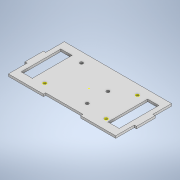
# Autodesk Inventor part: Level2 (Arduino)
Saved by Autodesk Inventor 2020 (Build 240168000, 168)
## iProperties
Created: 2020-01-30
Part Number: Level2 (Arduino)
Material: Generic
Document SubType Name: Modeling
Designer: jelte
Density: 1 g/cm^3
Appearance: Default
Mass: 27.7069 g
Surface Area: 213.533 cm^2
Volume: 27.7069 cm^3
Author: jelte
Autodesk Inventor part; units mm, degrees
ref_plane "YZ Plane" through (0, 0, 0) normal (1, 0, 0) x (0, 1, 0)
ref_plane "XZ Plane" through (0, 0, 0) normal (0, 1, 0) x (-1, 0, 0)
ref_plane "XY Plane" through (0, 0, 0) normal (0, 0, 1) x (1, 0, 0)
sketch "Sketch1" plane through (0, 0, 0) normal (0, 1, 0) x (-1, 0, 0)
  line L0 (71.1097, -38.0648) -> (71.1097, -13.0648)
  line L1 (71.1097, -13.0648) -> (74.1097, -13.0648)
  line L2 (74.1097, -13.0648) -> (74.1097, 11.9352)
  line L3 (74.1097, 11.9352) -> (71.1097, 11.9352)
  line L4 (71.1097, 11.9352) -> (71.1097, 36.9352)
  line L5 (-72.8903, -38.0648) -> (-72.8903, -13.0648)
  line L6 (-72.8903, 36.9352) -> (-72.8903, 11.9352)
  line L7 (-72.8903, -13.0648) -> (-75.8903, -13.0648)
  line L8 (-75.8903, -13.0648) -> (-75.8903, 11.9352)
  line L9 (-75.8903, 11.9352) -> (-72.8903, 11.9352)
  line L10 (71.1097, -38.0648) -> (-72.8903, -38.0648)
  line L11 (71.1097, 36.9352) -> (-72.8903, 36.9352)
  point P0 (0, 0)
  constraints: 24 end point, 5 perpendicular, 3 horizontal, 2 vertical
extrude "Extrusion1" add sketch "Sketch1" along normal blind 3
sketch "Sketch2" plane through (0, 3, 0) normal (0, 1, 0) x (1, 0, 0)
  line L0 (-74.1097, 13.0648) -> (-74.1097, -11.9352) projected
  line L1 (75.8903, -11.9352) -> (75.8903, 13.0648) projected
  line L2 (-71.1097, -36.9352) -> (72.8903, -36.9352) projected
  line L3 (-24.1097, -36.9352) -> (25.8903, -36.9352)
  line L4 (25.8903, -36.9352) -> (25.8903, -33.9352)
  line L5 (25.8903, -33.9352) -> (-24.1097, -33.9352)
  line L6 (-24.1097, -33.9352) -> (-24.1097, -36.9352)
  line L7 (72.8903, 38.0648) -> (-71.1097, 38.0648) projected
  point P0 (0, 0)
  dimension "d13" = 50
  dimension "d14" = 3
  constraints: 8 end point, 2 parallel, 1 horizontal, 1 perpendicular, 1 point on line
  measures "d13" distance of L4.end L5.end
  measures "d14" distance of L3.end L4.end
extrude "Extrusion2" cut sketch "Sketch2" against normal blind 30
sketch "Sketch3" plane through (0, 3, 0) normal (0, 1, 0) x (1, 0, 0)
  line L0 (-71.1097, -36.9352) -> (-24.1097, -36.9352) projected
  line L1 (-74.1097, 13.0648) -> (-74.1097, -11.9352) projected
  line L2 (-54.9097, 25.4648) -> (-64.9114, 25.4648)
  line L3 (-64.9114, 25.4648) -> (-64.9114, -24.8352)
  line L4 (-64.9114, -24.8352) -> (-54.9097, -24.8352)
  line L5 (-54.9097, -24.8352) -> (-54.9097, 25.4648)
  line L6 (56.6903, 25.4648) -> (66.6903, 25.4648)
  line L7 (66.6903, 25.4648) -> (66.6903, -24.8352)
  line L8 (66.6903, -24.8352) -> (56.6903, -24.8352)
  line L9 (56.6903, -24.8352) -> (56.6903, 25.4648)
  circle A0 centre (-34.6697, 22.9248) radius 2
  circle A1 centre (-35.9397, -22.2952) radius 2
  circle A2 centre (40.2603, 22.9248) radius 2
  circle A3 centre (46.6103, -22.2952) radius 2
  line L10 (-49.9097, 28.4648) -> (51.6903, 28.4648)
  line L11 (51.6903, 28.4648) -> (51.6903, 33.4648)
  line L12 (51.6903, 33.4648) -> (-49.9097, 33.4648)
  line L13 (-49.9097, 33.4648) -> (-49.9097, 28.4648)
  point P0 (0, 0)
  dimension "d32" = 4
  dimension "d35" = 4
  dimension "d38" = 4
  dimension "d39" = 4
  constraints: 24 end point, 6 parallel, 4 centre point, 3 horizontal, 3 perpendicular
  measures "d32" diameter of A0
  measures "d35" diameter of A1
  measures "d38" diameter of A2
  measures "d39" diameter of A3
extrude "Extrusion3" cut sketch "Sketch3" against normal blind 10
sketch "Sketch4" plane through (-49.9097, 3, -33.4648) normal (0, 0, 1) x (1, 0, 0)
  line L0 (0, 0) -> (101.6, 0) projected
  line L1 (0, 0) -> (101.6, 0)
  line L2 (101.6, 0) -> (101.6, -3)
  line L3 (101.6, -3) -> (0, -3)
  line L4 (0, -3) -> (0, 0)
  point P0 (49.9097, -3)
  constraints: 8 end point, 2 parallel, 1 horizontal, 1 perpendicular
extrude "Extrusion4" add sketch "Sketch4" along normal blind 5.2375
sketch "Sketch5" plane through (0, 3, 0) normal (0, 1, 0) x (1, 0, 0)
  circle A0 centre (-34.6697, 22.9248) radius 2 projected
  circle A1 centre (-34.6697, 22.9248) radius 2
  circle A2 centre (40.2603, 22.9248) radius 2 projected
  circle A3 centre (40.2603, 22.9248) radius 2
  circle A4 centre (46.6103, -22.2952) radius 2 projected
  circle A5 centre (46.6103, -22.2952) radius 2
  circle A6 centre (-35.9397, -22.2952) radius 2 projected
  circle A7 centre (-35.9397, -22.2952) radius 2
  point P0 (0, 0)
  constraints: 4 centre point, 4 coincident
extrude "Extrusion5" add sketch "Sketch5" against normal blind 3
sketch "Sketch6" plane through (0, 3, 0) normal (0, 1, 0) x (1, 0, 0)
  point P0 (0, 0)
sketch "Sketch7" plane through (0, 3, 0) normal (0, 1, 0) x (1, 0, 0)
  line L0 (-54.9097, -24.8352) -> (-54.9097, 25.4648) projected
  line L1 (56.6903, 25.4648) -> (56.6903, -24.8352) projected
  line L2 (72.8903, 38.0648) -> (-71.1097, 38.0648) projected
  line L3 (25.8903, -36.9352) -> (72.8903, -36.9352) projected
  line L4 (-74.1097, 13.0648) -> (-74.1097, -11.9352) projected
  line L5 (75.8903, -11.9352) -> (75.8903, 13.0648) projected
  line L6 (-64.9114, 25.4648) -> (-64.9114, -24.8352) projected
  line L7 (-64.9114, 25.4648) -> (-54.9097, 25.4648)
  line L8 (-54.9097, 25.4648) -> (-54.9097, 27.2348)
  line L9 (-54.9097, 27.2348) -> (-64.9114, 27.2348)
  line L10 (-64.9114, 27.2348) -> (-64.9114, 25.4648)
  line L11 (-64.9114, -24.8352) -> (-54.9097, -24.8352)
  line L12 (-54.9097, -24.8352) -> (-54.9097, -26.1052)
  line L13 (-54.9097, -26.1052) -> (-64.9114, -26.1052)
  line L14 (-64.9114, -26.1052) -> (-64.9114, -24.8352)
  line L15 (56.6903, -24.8352) -> (66.6903, -24.8352) projected
  line L16 (56.6903, -24.8352) -> (66.6903, -24.8352)
  line L17 (66.6903, -24.8352) -> (66.6903, -26.1052)
  line L18 (66.6903, -26.1052) -> (56.6903, -26.1052)
  line L19 (56.6903, -26.1052) -> (56.6903, -24.8352)
  line L20 (66.6903, 25.4648) -> (56.6903, 25.4648) projected
  line L21 (56.6903, 25.4648) -> (66.6903, 25.4648)
  line L22 (66.6903, 25.4648) -> (66.6903, 27.2348)
  line L23 (66.6903, 27.2348) -> (56.6903, 27.2348)
  line L24 (56.6903, 27.2348) -> (56.6903, 25.4648)
  circle A0 centre (-35.9397, -23.5652) radius 2
  circle A1 centre (46.6103, -23.5652) radius 2
  circle A2 centre (-34.6697, 24.6948) radius 2
  circle A3 centre (40.2603, 24.6948) radius 2
  circle A4 centre (16.1303, -18.4852) radius 2
  circle A5 centre (16.1303, 9.4148) radius 2
  point P0 (0, 0)
  dimension "d61" = 4
  dimension "d63" = 4
  dimension "d69" = 4
  dimension "d71" = 4
  dimension "d74" = 4
  dimension "d76" = 4
  constraints: 32 end point, 8 parallel, 6 centre point, 4 horizontal, 4 perpendicular, 4 point on line
  measures "d61" diameter of A0
  measures "d63" diameter of A1
  measures "d69" diameter of A2
  measures "d71" diameter of A3
  measures "d74" diameter of A4
  measures "d76" diameter of A5
extrude "Extrusion6" cut sketch "Sketch7" against normal blind 3 contours L12 L13 L14 L11 | L7 L10 L9 L8 | L15 L17 L18 L19 | L24 L23 L22 L20 | A0 | A1 | A2 | A3 | A4 | A5
sketch "Sketch8" plane through (0, 3, 0) normal (0, 1, 0) x (1, 0, 0)
  point P0 (0, 0)
sketch "Sketch9" plane through (0, 3, 0) normal (0, 1, 0) x (1, 0, 0)
  circle A0 centre (46.6103, -23.5652) radius 2 projected
  circle A1 centre (-35.9397, -23.5652) radius 2 projected
  circle A2 centre (40.2603, 24.6948) radius 2 projected
  point P0 (0, 0)
sketch "Sketch10" plane through (0, 3, 0) normal (0, 1, 0) x (1, 0, 0)
  line L0 (56.6903, 27.2348) -> (66.6903, 27.2348) projected
  line L1 (56.6903, 27.2348) -> (51.6903, 27.2348)
  line L2 (51.6903, 27.2348) -> (51.6903, -26.1052)
  line L3 (51.6903, -26.1052) -> (56.6903, -26.1052)
  line L4 (56.6903, -26.1052) -> (56.6903, 27.2348)
  line L5 (-54.9097, -26.1052) -> (-54.9097, 27.2348) projected
  line L6 (-54.9097, 27.2348) -> (-49.9097, 27.2348)
  line L7 (-49.9097, 27.2348) -> (-49.9097, -26.1052)
  line L8 (-49.9097, -26.1052) -> (-54.9097, -26.1052)
  line L9 (-54.9097, -26.1052) -> (-54.9097, 27.2348)
  point P0 (0, 0)
  dimension "d79" = 5
  dimension "d80" = 5
  constraints: 16 end point, 4 parallel, 2 horizontal, 2 perpendicular
  measures "d79" distance of L0.start L1.end
  measures "d80" distance of L5.end L6.end
extrude "Extrusion7" cut sketch "Sketch10" against normal blind 10
body "Solid1"
